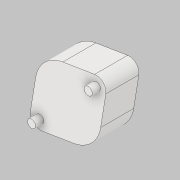
# Autodesk Inventor part: Caster_wheel_inner_plug_1_02
Saved by Autodesk Inventor 2019.3 (Build 233278000, 278)
## iProperties
Created: 2019-03-27
Part Number: Caster_wheel_inner_plug_1_02
Material: Generic
Document SubType Name: Modeling
Designer: Varga Daniel
Density: 1 g/cm^3
Appearance: White - P 1-1 C
Author: Varga Daniel
Autodesk Inventor part; units mm, degrees
ref_plane "YZ Plane" through (0, 0, 0) normal (1, 0, 0) x (0, 1, 0)
ref_plane "XZ Plane" through (0, 0, 0) normal (0, 1, 0) x (-1, 0, 0)
ref_plane "Work Plane2" through (0, 0, 0) normal (0, 0, 1) x (1, 0, 0)
sketch "Sketch1" plane through (0, 0, 0) normal (0, 0, 1) x (1, 0, 0)
  circle A0 centre (-28.0566, -29.4795) radius 1.95
  circle A1 centre (-0.5502, -1.973) radius 1.95
  arc A2 (3.9968, -2.877) -> (-1.4542, 2.574) centre (-0.6916, -2.1144) ccw
  line L0 (1.4891, -18.2949) -> (3.9968, -2.877)
  arc A3 (-11.7347, -31.5187) -> (1.4891, -18.2949) centre (-14.3034, -15.7262) ccw
  line L1 (-27.1526, -34.0264) -> (-11.7347, -31.5187)
  arc A4 (-32.6036, -28.5755) -> (-27.1526, -34.0264) centre (-27.9152, -29.338) ccw
  line L2 (-30.0959, -13.1576) -> (-32.6036, -28.5755)
  arc A5 (-16.8721, 0.0662) -> (-30.0959, -13.1576) centre (-14.3034, -15.7262) ccw
  line L3 (-1.4542, 2.574) -> (-16.8721, 0.0662)
  circle A6 centre (-9.3034, -10.7262) radius 2.5
  circle A7 centre (-19.3034, -10.7262) radius 2.5
  circle A8 centre (-9.3034, -20.7262) radius 2.5
  circle A9 centre (-19.3034, -20.7262) radius 2.5
  circle A10 centre (-9.3034, -10.7262) radius 2.4
  circle A11 centre (-9.3034, -20.7262) radius 2.4
  circle A12 centre (-19.3034, -20.7262) radius 2.4
  circle A13 centre (-19.3034, -10.7262) radius 2.4
  line L4 (-0.6916, -2.1144) -> (-27.9152, -29.338) construction
  line L5 (-14.3034, -15.7262) -> (-12.5748, -17.4548) construction
  point P0 (0, 0)
  dimension "d2" = 0.1
  dimension "d3" = 0.1
  dimension "d4" = 0.1
  dimension "d5" = 0.1
  dimension "d10" = 3.9
  dimension "d11" = 3.9
  dimension "d12" = 38.7
  constraints: 14 centre point, 12 end point, 8 point on circle, 1 perpendicular, 1 symmetric about line, 2 other
  measures "d2" radial gap between concentric circles of A6 A10
  measures "d3" radial gap between concentric circles of A8 A11
  measures "d4" radial gap between concentric circles of A9 A12
  measures "d5" radial gap between concentric circles of A7 A13
  measures "d10" diameter of A0
  measures "d11" diameter of A1
  measures "d12" distance of A0.centre L4.start
extrude "Extrusion1" add sketch "Sketch1" along normal blind 16.03 contours A0 | A1 | L0 A3 L1 A4 L2 A5 L3 A2 | A6 | A7 | A8 | A9 | A10 | A11 | A12 | A13
extrude "Extrusion2" add sketch "Sketch1" against normal blind 9.2 contours A10 | A11 | A12 | A13
extrude "Extrusion3" add sketch "Sketch1" along normal blind 20.03 contours A0 | A1
equation "\"d10\" = d11"
equation "\"d0\" = inner_plug_height"
equation "\"inner_plug_height\" = 16.03"
body "Solid1"
